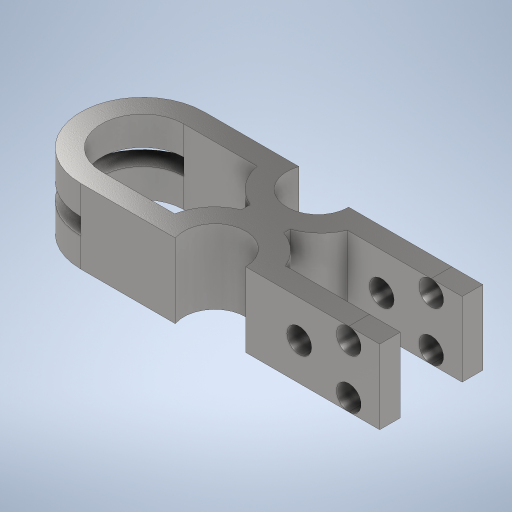
# Autodesk Inventor part: drawing
Saved by Autodesk Inventor 2024 (Build 280153000, 153)
## iProperties
Created: 2024-02-02
Part Number: drawing
Material: Stahl, galvanisiert
Document SubType Name: Modeling
Designer: ffogue
Density: 7.85 g/cm^3
Appearance: Galvanisiert
Author: ffogue
Autodesk Inventor part; units mm, degrees
ref_plane "YZ Plane" through (0, 0, 0) normal (1, 0, 0) x (0, 1, 0)
ref_plane "XZ Plane" through (0, 0, 0) normal (0, 1, 0) x (-1, 0, 0)
sketch "Skizze1" plane through (0, 0, 0) normal (0, 0, 1) x (1, 0, 0)
  line L0 (75, 25) -> (140, 25)
  line L1 (140, -25) -> (75, -25)
  line L2 (140, 15) -> (84.3835, 15)
  line L3 (140, -15) -> (84.3835, -15)
  line L4 (175.9728, 0) -> (38.8128, 0) construction
  line L5 (75, 25) -> (75, -25) construction
  arc A0 (70, 1.5) -> (84.3835, 15) centre (61.4706, 25) ccw
  line L6 (70, 1.5) -> (70, -1.5)
  arc A1 (84.3835, -15) -> (70, -1.5) centre (61.4706, -25) ccw
  line L7 (140, 25) -> (140, 15)
  line L8 (140, -15) -> (140, -25)
  arc A2 (45.8579, 30) -> (75, 25) centre (60, 25) ccw
  line L9 (45.8579, 30) -> (0, 30)
  arc A3 (75, -25) -> (45.8579, -30) centre (60, -25) ccw
  line L10 (45.8579, -30) -> (0, -30)
  arc A4 (0, 30) -> (0, -30) centre (0, 0) ccw
  line L11 (50, 2.0871) -> (50, -2.0871)
  line L12 (35.5051, -20) -> (0, -20)
  line L13 (35.5051, 20) -> (0, 20)
  arc A5 (0, 20) -> (0, -20) centre (0, 0) ccw
  line L14 (60, 25) -> (60, -25) construction
  arc A6 (35.5051, 20) -> (50, 2.0871) centre (60, 25) ccw
  arc A7 (50, -2.0871) -> (35.5051, -20) centre (60, -25) ccw
  dimension "d17" = 30
  dimension "d18" = 50
  dimension "d19" = 25
  dimension "d20" = 3
  dimension "d21" = 80
  dimension "d28" = 15
  dimension "d30" = 30
  dimension "d34" = 20
  dimension "d36" = 25
  dimension "d37" = 25
  dimension "d38" = 60
  dimension "d39" = 20
  constraints: 30 end point, 16 point on circle, 8 centre point, 6 tangent, 5 horizontal, 5 perpendicular, 4 parallel, 3 horizontal alignment, 3 symmetric about line, 2 coincident, 1 concentric, 1 equal radius, 1 point on line, 1 vertical, 1 vertical alignment, 4 other
  measures "d17" distance between parallel lines of L3 L2
  measures "d18" distance between parallel lines of L1 L0
  measures "d19" radius of A1
  measures "d20" distance of L6.start L6.end
  measures "d21" distance from line of L7 L14.start
  measures "d28" radius of A2
  measures "d30" radius of A4
  measures "d34" distance between parallel lines of L6 L11
  measures "d36" radius of A7
  measures "d37" radius of A6
  measures "d38" horizontal distance of L14.start point (0, 0)
  measures "d39" radius of A5
extrude "Extrusion1" add sketch "Skizze1" along normal blind 36
sketch "Skizze2" plane through (75, 25, 0) normal (0, 1, 0) x (1, 0, 0)
  line L0 (65, 0) -> (65, -36) projected
  line L1 (65, 0) -> (0, 0) projected
  point P0 (-75, 0)
  point P1 (50, -6)
  point P2 (50, -30)
  point P3 (26, -18)
  point P4 (65, -18)
  dimension "d42" = 24
  dimension "d43" = 6
  dimension "d44" = 24
  dimension "d45" = 15
  constraints: 1 horizontal alignment, 1 midpoint, 1 vertical alignment
  measures "d42" distance of point (50, -30) point (50, -6)
  measures "d43" distance from line of point (50, -6) L1
  measures "d44" horizontal distance of point (50, -6) point (26, -18)
  measures "d45" distance from line of L0 point (50, -6)
hole "Bohrung1" at (125, 25, 6) at (125, 25, 30) at (101, 25, 18) direction (0, -1, 0) diameter 12 depth 50
ref_plane "Arbeitsebene1" through (0, 0, 18) normal (0, 0, 1) x (1, 0, 0)
sketch "Skizze3" plane through (0, 0, 18) normal (0, 0, 1) x (1, 0, 0)
  arc A0 (0, 30) -> (0, -30) centre (0, 0) ccw projected
  arc A1 (0, 30) -> (0, -30) centre (0, 0) ccw
  line L0 (0, -30) -> (0, 30)
  dimension "d54" = 30
  constraints: 2 end point, 2 point on circle, 1 centre point, 1 vertical
  measures "d54" radius of A0
extrude "Extrusion2" cut sketch "Skizze3" along normal mid plane 8
equation "\"d37\" = d36"
